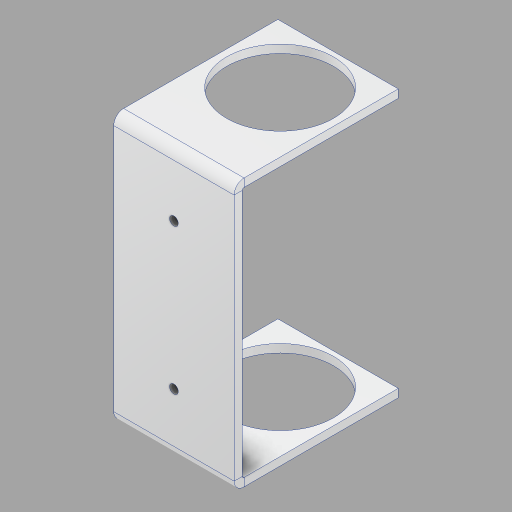
# Autodesk Inventor part: servo_horn_bracket_test
Saved by Autodesk Inventor 2023.1 (Build 271208000, 208)
## iProperties
Created: 2022-10-18
Part Number: servo_horn_bracket_test
Material: 알루미늄 6061
Document SubType Name: Sheet Metal
Designer: 박동준
Density: 2.7 g/cm^3
Sheet Metal Rule: 기본값_mm
Appearance: 알루미늄 - 평지
Author: 박동준
Autodesk Inventor part; units mm, degrees
ref_plane "YZ Plane" through (0, 0, 0) normal (1, 0, 0) x (0, 1, 0)
ref_plane "XZ Plane" through (0, 0, 0) normal (0, 1, 0) x (-1, 0, 0)
ref_plane "XY Plane" through (0, 0, 0) normal (0, 0, 1) x (1, 0, 0)
sketch "스케치1" plane through (0, 0, 0) normal (0, 0, 1) x (1, 0, 0)
  line L0 (-11, 24.45) -> (11, 24.45)
  line L1 (11, 24.45) -> (11, -24.45)
  line L2 (11, -24.45) -> (-11, -24.45)
  line L3 (-11, -24.45) -> (-11, 24.45)
  point P0 (0, 0)
  point P1 (0, 24.45)
  point P2 (-11, 0)
  dimension "d0" = 22
  dimension "d1" = 48.9
  measures "d0" distance of L0.start L0.end
  measures "d1" distance of L2.end L0.start
extrude "판1" add sketch "스케치1" along normal mid plane 1.5
sketch "스케치2" plane through (11, 22.95, 0.75) normal (0, 1, 0) x (-1, 0, 0)
  line L0 (22, 0) -> (0, 0)
  line L1 (0, 0) -> (0, -30)
  line L2 (0, -30) -> (22, -30)
  line L3 (22, -30) -> (22, 0)
  constraints: 6 end point, 1 horizontal, 1 perpendicular, 1 vertical
edge flange "플랜지1" height 30 angle 90 thickness 1.5 bend radius 0.31 thickness toward (0, 1, 0) relief tear relief width 1.5 relief depth 0.75 corner gap 0.31 corner form 0 edges at (0, 24.45, -0.75) (0, -24.45, -0.75) wall of the first edge with corners at (-11, 22.95, 0.75) (11, 22.95, 0.75) (11, 22.95, -29.25) (-11, 22.95, -29.25)
bend "절곡부1"
corner "구석1"
sketch "스케치3" plane through (-11, 24.45, -29.25) normal (0, 1, 0) x (1, 0, 0)
  circle A0 centre (11, -10.595) radius 9.75
  line L0 (0, -28.19) -> (0, 0) projected
  line L1 (0, 0) -> (22, 0) projected
  point P0 (11, -29.25)
  point P1 (0, -14.095)
  point P2 (11, 0)
  dimension "d13" = 19.5
  dimension "d32" = 10.595
  constraints: 2 midpoint, 1 centre point, 1 vertical alignment
  measures "d13" diameter of A0
  measures "d32" distance from line of L1 A0.centre
extrude "돌출1" cut sketch "스케치3" against normal through all
sketch "스케치4" plane through (0, 0, 0.75) normal (0, 0, 1) x (1, 0, 0)
  circle A0 centre (0, 13.05) radius 1.05
  circle A1 centre (0, -13.55) radius 1.05
  line L0 (11, 22.64) -> (-11, 22.64) projected
  line L1 (-11, -22.64) -> (11, -22.64) projected
  point P0 (0, 0)
  dimension "d16" = 2.1
  dimension "d17" = 2.1
  dimension "d18" = 9.59
  dimension "d31" = 9.09
  constraints: 2 centre point, 2 coincident, 2 vertical alignment
  measures "d16" diameter of A0
  measures "d17" diameter of A1
  measures "d18" distance from line of L0 A0.centre
  measures "d31" distance from line of L1 point (0, -13.55)
hole "구멍1" at (0, 13.05, 0.75) at (0, -13.55, 0.75) direction (0, 0, -1) diameter 1.567 end through all thread size "M2x0.4" class "6H" standard "ISO Metric profile"
equation "\"TransitionRadius\" = BendRadius"
